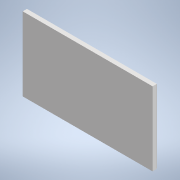
# Autodesk Inventor part: TV
Saved by Autodesk Inventor 2020 (Build 240168000, 168)
## iProperties
Created: 2020-02-25
Part Number: TV
Material: Generic
Document SubType Name: Modeling
Designer: Patrik
Density: 1 g/cm^3
Appearance: Default
Author: Patrik
Autodesk Inventor part; units mm, degrees
ref_plane "YZ Plane" through (0, 0, 0) normal (1, 0, 0) x (0, 1, 0)
ref_plane "XZ Plane" through (0, 0, 0) normal (0, 1, 0) x (-1, 0, 0)
ref_plane "XY Plane" through (0, 0, 0) normal (0, 0, 1) x (1, 0, 0)
sketch "Sketch1" plane through (0, 0, 0) normal (0, 0, 1) x (1, 0, 0)
  line L0 (0, 0) -> (1684, 0)
  line L1 (1684, 0) -> (1684, 955)
  line L2 (1684, 955) -> (0, 955)
  line L3 (0, 955) -> (0, 0)
  dimension "d0" = 1684
  dimension "d1" = 955
  constraints: 8 end point, 2 parallel, 1 horizontal, 1 perpendicular
  measures "d0" distance of L2.end L1.end
  measures "d1" distance of L1.end L0.end
extrude "Extrusion1" add sketch "Sketch1" along normal blind 61
fillet "Fillet1" radius 10 4 edges at (0, 477.5, 0) (842, 955, 0) (842, 0, 0) (1684, 477.5, 0)
sketch "Sketch2" plane through (0, 0, 0) normal (0, 0, -1) x (-1, 0, 0)
  point P0 (0, 0)
sketch "Sketch3" plane through (0, 0, 0) normal (0, 0, -1) x (-1, 0, 0)
  line L0 (-1658.1713, 929.1713) -> (-29.133, 929.1713)
  line L1 (-29.133, 929.1713) -> (-29.133, 29.4852)
  line L2 (-29.133, 29.4852) -> (-1658.1713, 29.4852)
  line L3 (-1658.1713, 29.4852) -> (-1658.1713, 929.1713)
  point P0 (0, 0)
  constraints: 8 end point, 2 parallel, 1 horizontal, 1 perpendicular
extrude "Extrusion2" cut sketch "Sketch3" against normal blind 5
body "Solid1"
